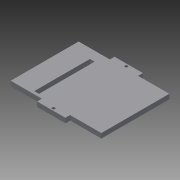
# Autodesk Inventor part: face
Saved by Autodesk Inventor 2014 (Build 180170000, 170)
## iProperties
Created: 2014-03-02
Part Number: face
Material: 常规
Document SubType Name: Modeling
Designer: Keshuai
Density: 1 g/cm^3
Appearance: 默认
Author: Keshuai
Autodesk Inventor part; units mm, degrees
ref_plane "YZ Plane" through (0, 0, 0) normal (1, 0, 0) x (0, 1, 0)
ref_plane "XZ Plane" through (0, 0, 0) normal (0, 1, 0) x (-1, 0, 0)
ref_plane "XY Plane" through (0, 0, 0) normal (0, 0, 1) x (1, 0, 0)
sketch "草图1" plane through (0, 0, 0) normal (0, 0, 1) x (1, 0, 0)
  line L0 (33, 0) -> (46.5, 0) projected
  line L1 (33, 5) -> (46.5, 5) projected
  line L2 (25, -72) -> (33, -72) projected
  line L3 (0, 0) -> (96, 0)
  line L4 (96, 0) -> (96, -72)
  line L5 (96, -72) -> (0, -72)
  line L6 (0, -72) -> (0, 0)
  line L7 (27, -69) -> (22, -69)
  line L8 (22, -69) -> (22, -10)
  line L9 (22, -10) -> (27, -10)
  line L10 (27, -10) -> (27, -69)
  line L11 (48, -81.8349) -> (48, 25.2825) construction
  line L12 (33, 0) -> (63, 0)
  line L13 (63, 0) -> (63, 5)
  line L14 (63, 5) -> (33, 5)
  line L15 (33, 5) -> (33, 0)
  line L16 (33, 0) -> (63, 5) construction
  line L17 (63, 0) -> (33, 5) construction
  line L18 (46, -77) -> (61, -77) projected
  line L19 (63, -72) -> (33, -72)
  line L20 (33, -72) -> (33, -77)
  line L21 (33, -77) -> (63, -77)
  line L22 (63, -77) -> (63, -72)
  circle A0 centre (48, 2.5) radius 1.5
  circle A1 centre (48, -74.5) radius 1.5
  line L23 (33, 5) -> (33, 0) projected
  line L24 (46.5, 0) -> (46.5, 5) projected
  dimension "d0" = 3
  dimension "d1" = 10
  dimension "d2" = 59
  dimension "d3" = 5
  dimension "d4" = 22
  dimension "d6" = 3
  dimension "d7" = 3
  constraints: 38 end point, 9 parallel, 5 point on line, 4 horizontal, 4 perpendicular, 3 collinear, 2 centre point, 2 midpoint, 1 coincident
  measures "d0" distance between parallel lines of L5 L7
  measures "d1" distance between parallel lines of L0 L9
  measures "d2" distance between parallel lines of L9 L7
  measures "d3" distance between parallel lines of L10 L8
  measures "d4" distance between parallel lines of L6 L8
  measures "d6" diameter of A0
  measures "d7" diameter of A1
extrude "拉伸1" add sketch "草图1" along normal blind 5
